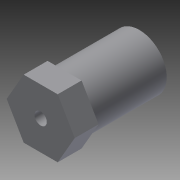
# Autodesk Inventor part: Part1
Saved by Autodesk Inventor 2016 (Build 200138000, 138)
## iProperties
Created: 2015-05-23
Part Number: Part1
Material: Generic
Document SubType Name: Modeling
Designer: Jufo
Density: 1 g/cm^3
Appearance: Default
Author: Jufo
Autodesk Inventor part; units mm, degrees
ref_plane "YZ Plane" through (0, 0, 0) normal (1, 0, 0) x (0, 1, 0)
ref_plane "XZ Plane" through (0, 0, 0) normal (0, 1, 0) x (-1, 0, 0)
ref_plane "XY Plane" through (0, 0, 0) normal (0, 0, 1) x (1, 0, 0)
sketch "Sketch1" plane through (0, 0, 0) normal (0, 1, 0) x (-1, 0, 0)
  line L0 (6.825, 0) -> (3.4125, -5.9106)
  line L1 (3.4125, -5.9106) -> (-3.4125, -5.9106)
  line L2 (-3.4125, -5.9106) -> (-6.825, 0)
  line L3 (-6.825, 0) -> (-3.4125, 5.9106)
  line L4 (-3.4125, 5.9106) -> (3.4125, 5.9106)
  line L5 (3.4125, 5.9106) -> (6.825, 0)
  point P0 (0, 0)
  point P1 (0, 0)
  dimension "d1" = 13.65
  constraints: 12 end point, 1 coincident, 13 other
  measures "d1" distance of L0.start L2.end
extrude "Extrusion1" add sketch "Sketch1" along normal blind 4.8
sketch "Sketch2" plane through (0, 4.8, 0) normal (0, 1, 0) x (1, 0, 0)
  circle A0 centre (0, 0) radius 5.5
  circle A1 centre (0, 0) radius 1.625
  line L0 (-1.1726, 1.125) -> (1.1726, 1.125)
  line L1 (0, -1.625) -> (0, 1.125)
  dimension "d4" = 11
  dimension "d5" = 3.25
  dimension "d56" = 2.75
  constraints: 4 end point, 3 point on circle, 2 centre point, 2 coincident, 1 midpoint
  measures "d4" diameter of A0
  measures "d5" diameter of A1
  measures "d56" distance of L1.start L1.end
extrude "Extrusion2" add sketch "Sketch2" along normal blind 15 contours A0 | L0 A1
sketch "Sketch7" plane through (-1.1726, 19.8, -1.125) normal (0, 0, 1) x (1, 0, 0)
  line L0 (0, 0) -> (2.3452, 0) projected
  line L1 (0, -15) -> (0, 0) projected
  line L2 (1.1726, 0) -> (1.1726, -3)
  circle A0 centre (1.1726, -3) radius 1
  point P0 (0, -0.5)
  point P1 (1.1726, -19.8)
  dimension "d33" = 3
  dimension "d34" = 2
  constraints: 2 end point, 1 centre point, 1 coincident, 1 midpoint, 1 parallel
  measures "d33" distance of L2.start L2.end
  measures "d34" diameter of A0
hole "Hole1" at (0, 16.8, -1.125) direction (0, 0, -1) diameter 2.1 depth 8 tip angle 118
sketch "Sketch8" plane through (0, 0, 0) normal (0, -1, 0) x (1, 0, 0)
  circle A0 centre (0, 0) radius 1.5
  dimension "d42" = 3
  constraints: 1 centre point, 1 coincident
  measures "d42" diameter of A0
hole "Hole2" at (0, 0, 0) direction (0, 1, 0) diameter 2.459 depth 7 tip angle 118
sketch "Sketch10" plane through (0, 19.8, 0) normal (0, 1, 0) x (1, 0, 0)
  circle A0 centre (0, 0) radius 5.5 projected
  line L0 (3.4293, 4.3) -> (-3.4293, 4.3)
  line L1 (0, 5.5) -> (0, 4.3)
  dimension "d60" = 1.2
  constraints: 4 end point, 3 point on circle, 1 midpoint
  measures "d60" distance of L1.start L1.end
extrude "Extrusion7" cut sketch "Sketch10" against normal blind 6 contours L0 L1 A0 | A0 L1 L0
body "Solid1"
